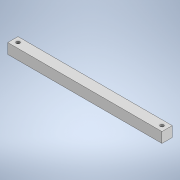
# Autodesk Inventor part: レール
Saved by Autodesk Inventor 2022 (Build 260153070, 153G)
## iProperties
Created: 2022-10-10
Part Number: レール
Material: 一般
Document SubType Name: Modeling
Designer: hirok
Density: 1 g/cm^3
Appearance: 既定
Author: hirok
Autodesk Inventor part; units mm, degrees
ref_plane "YZ Plane" through (0, 0, 0) normal (1, 0, 0) x (0, 1, 0)
ref_plane "XZ Plane" through (0, 0, 0) normal (0, 1, 0) x (-1, 0, 0)
ref_plane "XY Plane" through (0, 0, 0) normal (0, 0, 1) x (1, 0, 0)
sketch "スケッチ1" plane through (0, 0, 0) normal (0, 0, 1) x (1, 0, 0)
  line L0 (0, 0) -> (150, 0)
  line L1 (150, 0) -> (150, 10)
  line L2 (150, 10) -> (0, 10)
  line L3 (0, 10) -> (0, 0)
  dimension "d0" = 10
  dimension "d1" = 150
  constraints: 8 end point, 2 parallel, 1 horizontal, 1 perpendicular
  measures "d0" distance between parallel lines of L0 L2
  measures "d1" distance of L0.start L0.end
extrude "押し出し1" add sketch "スケッチ1" along normal blind 10
sketch "スケッチ2" plane through (0, 10, 0) normal (0, 1, 0) x (1, 0, 0)
  line L0 (150, 0) -> (0, 0) projected
  line L1 (0, 0) -> (0, -10) projected
  line L2 (75, 0) -> (75, -10)
  line L3 (150, -10) -> (0, -10) projected
  point P0 (5, -5)
  point P1 (145, -5)
  dimension "d4" = 5
  dimension "d5" = 5
  constraints: 2 end point, 2 midpoint, 1 symmetric about line
  measures "d4" distance from line of point (5, -5) L0
  measures "d5" distance from line of L1 point (5, -5)
hole "穴1" at (5, 10, 5) at (145, 10, 5) direction (0, -1, 0) diameter 3.4 end through all clearance for "Countersunk Flat Head Screw ISO 2009/7046" size "M3" standard "ISO"
